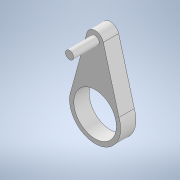
# Autodesk Inventor part: ClickSpringBacking
Saved by Autodesk Inventor 2021 (Build 250183000, 183)
## iProperties
Created: 2021-07-10
Part Number: ClickSpringBacking
Material: Generic
Document SubType Name: Modeling
Designer: teh18
Density: 1 g/cm^3
Appearance: Default
Author: teh18
Autodesk Inventor part; units mm, degrees
ref_plane "YZ Plane" through (0, 0, 0) normal (1, 0, 0) x (0, 1, 0)
ref_plane "XZ Plane" through (0, 0, 0) normal (0, 1, 0) x (-1, 0, 0)
ref_plane "XY Plane" through (0, 0, 0) normal (0, 0, 1) x (1, 0, 0)
sketch "Sketch1" plane through (0, 0, 0) normal (0, 0, 1) x (1, 0, 0)
  circle A0 centre (0, 0) radius 3.75 projected
  circle A1 centre (0, 0) radius 15 projected
  arc A2 (-0.5916, -14.9883) -> (-0.5916, -14.9883) centre (0, 0) ccw
  circle A3 centre (0, 30.4603) radius 5
  circle A4 centre (0, 0) radius 12.5
  line L0 (4.7233, 32.1006) -> (14.0107, 5.3571)
  line L1 (-14.0107, 5.3571) -> (-4.7233, 32.1006)
  point P0 (-13.5955, 6.3373)
  point P1 (13.5955, 6.3373)
  point P2 (0.4183, 30.4603)
  dimension "d0" = 30
  dimension "d3" = 10
  dimension "d8" = 25
  constraints: 6 point on circle, 4 end point, 3 centre point, 2 tangent, 1 coincident, 1 vertical alignment
  measures "d0" diameter of A2
  measures "d3" diameter of A3
  measures "d8" diameter of A4
extrude "Extrusion1" add sketch "Sketch1" along normal blind 9 contours A1 | A1 L1 A3 L0 | A3
sketch "Sketch2" plane through (0, 0, 9) normal (0, 0, 1) x (1, 0, 0)
  circle A0 centre (0, 30.4603) radius 2.4
  circle A1 centre (0, 30.4603) radius 12
  line L0 (44.6109, 21.6834) -> (46.2306, 21.859) projected
  line L1 (48.8318, 20.2765) -> (49.4206, 18.7572) projected
  line L2 (49.4206, 18.7572) -> (50.4418, 20.0268) projected
  line L3 (53.3999, 20.7473) -> (54.8905, 20.0894) projected
  line L4 (54.8905, 20.0894) -> (54.7149, 21.7093) projected
  line L5 (56.2973, 24.3107) -> (57.8164, 24.8996) projected
  line L6 (57.8164, 24.8996) -> (56.5469, 25.9209) projected
  line L7 (55.8266, 28.8794) -> (56.4844, 30.3701) projected
  line L8 (56.4844, 30.3701) -> (54.8646, 30.1945) projected
  line L9 (52.2635, 31.777) -> (51.6747, 33.2963) projected
  line L10 (51.6747, 33.2963) -> (50.6535, 32.0266) projected
  line L11 (47.6953, 31.3062) -> (46.2048, 31.9641) projected
  line L12 (46.2048, 31.9641) -> (46.3804, 30.3441) projected
  line L13 (44.798, 27.7427) -> (43.2789, 27.1539) projected
  line L14 (43.2789, 27.1539) -> (44.5484, 26.1326) projected
  line L15 (45.2687, 23.1741) -> (44.6109, 21.6834) projected
  ellipse E0 centre (50.5476, 26.0267) end of major axis (50.311, 20.0305) minor radius 6.0002 (46.2306, 21.859) -> (48.8318, 20.2765) ccw projected
  ellipse E1 centre (50.5476, 26.0267) end of major axis (50.7843, 32.0229) minor radius 6.0002 (50.4418, 20.0268) -> (53.3999, 20.7473) ccw projected
  ellipse E2 centre (50.5476, 26.0267) end of major axis (50.7843, 32.0229) minor radius 6.0002 (54.7149, 21.7093) -> (56.2973, 24.3107) ccw projected
  ellipse E3 centre (50.5476, 26.0267) end of major axis (50.7843, 32.0229) minor radius 6.0002 (56.5469, 25.9209) -> (55.8266, 28.8794) ccw projected
  ellipse E4 centre (50.5476, 26.0267) end of major axis (50.7843, 32.0229) minor radius 6.0002 (54.8646, 30.1945) -> (52.2635, 31.777) ccw projected
  ellipse E5 centre (50.5476, 26.0267) end of major axis (50.311, 20.0305) minor radius 6.0002 (50.6535, 32.0266) -> (47.6953, 31.3062) ccw projected
  ellipse E6 centre (50.5476, 26.0267) end of major axis (50.311, 20.0305) minor radius 6.0002 (46.3804, 30.3441) -> (44.798, 27.7427) ccw projected
  ellipse E7 centre (50.5476, 26.0267) end of major axis (50.311, 20.0305) minor radius 6.0002 (44.5484, 26.1326) -> (45.2687, 23.1741) ccw projected
  ellipse E8 centre (50.5476, 26.0267) end of major axis (51.2575, 44.0127) minor radius 17.9981 projected
  arc A2 (4.7233, 32.1006) -> (-4.7233, 32.1006) centre (0, 30.4603) ccw projected
  point P0 (0, 0)
  dimension "d4" = 4.8
  dimension "d7" = 24
  constraints: 3 coincident, 2 centre point, 8 other
  measures "d4" diameter of A0
  measures "d7" diameter of A1
extrude "Extrusion2" add sketch "Sketch2" along normal blind 15 contours A0
body "Solid1"
